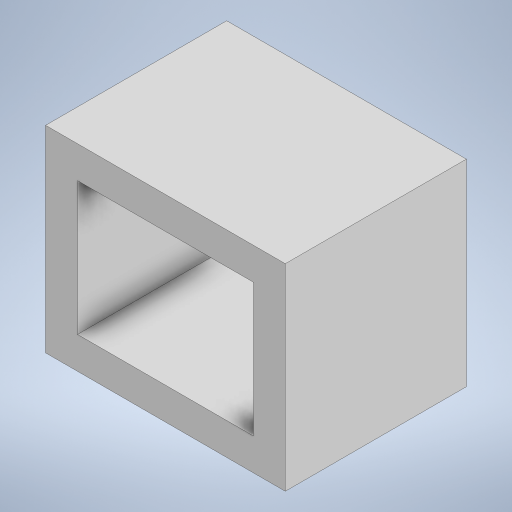
# Autodesk Inventor part: bracket_square_bottom
Saved by Autodesk Inventor 2024 (Build 280153000, 153)
## iProperties
Created: 2024-02-12
Part Number: bracket_square_bottom
Material: Generic
Document SubType Name: Modeling
Designer: clbri
Density: 1 g/cm^3
Appearance: Default
Author: clbri
Autodesk Inventor part; units mm, degrees
ref_plane "YZ Plane" through (0, 0, 0) normal (1, 0, 0) x (0, 1, 0)
ref_plane "XZ Plane" through (0, 0, 0) normal (0, 1, 0) x (-1, 0, 0)
ref_plane "XY Plane" through (0, 0, 0) normal (0, 0, 1) x (1, 0, 0)
sketch "Sketch1" plane through (0, 0, 0) normal (0, 0, 1) x (1, 0, 0)
  line L0 (0, 0) -> (16.5, 0)
  line L1 (16.5, 0) -> (16.5, 12.5)
  line L2 (16.5, 12.5) -> (0, 12.5)
  line L3 (0, 12.5) -> (0, 0)
  line L4 (-3, -3) -> (19.5, -3)
  line L5 (19.5, -3) -> (19.5, 15.5)
  line L6 (19.5, 15.5) -> (-3, 15.5)
  line L7 (-3, 15.5) -> (-3, -3)
  dimension "d0" = 16.5
  dimension "d1" = 12.5
  dimension "d2" = 22.5
  dimension "d3" = 3
  dimension "d4" = 3
  dimension "d5" = 3
  constraints: 16 end point, 4 parallel, 2 horizontal, 2 perpendicular
  measures "d0" distance of L2.end L1.end
  measures "d1" distance of L1.end L0.end
  measures "d2" distance of L6.end L5.end
  measures "d3" distance between parallel lines of L5 L1
  measures "d4" distance between parallel lines of L6 L2
  measures "d5" distance between parallel lines of L4 L0
extrude "Extrusion1" add sketch "Sketch1" along normal blind 17
body "Solid1"
